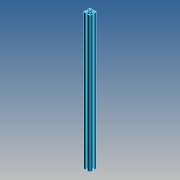
# Autodesk Inventor part: P100
Saved by Autodesk Inventor 2019 (Build 230136000, 136)
## iProperties
Created: 2016-06-02
Part Number: P100
Material: Aluminium
Document SubType Name: Modeling
Designer: serge.amoos
Density: 2.7 g/cm^3
Appearance: Sky Blue Dark
Description: Colonne
Author: serge.amoos
Autodesk Inventor part; units mm, degrees
ref_plane "YZ Plane" through (0, 0, 0) normal (1, 0, 0) x (0, 1, 0)
ref_plane "XZ Plane" through (0, 0, 0) normal (0, 1, 0) x (-1, 0, 0)
ref_plane "XY Plane" through (0, 0, 0) normal (0, 0, 1) x (1, 0, 0)
sketch "Sketch1" plane through (0, 0, 0) normal (0, 0, 1) x (1, 0, 0)
  line L0 (-24, 0) -> (4, 0) construction
  line L1 (0, -4) -> (0, 24) construction
  line L2 (0, 0) -> (-20, 20)
  line L3 (-20, 20) -> (0, 20)
  line L4 (0, 20) -> (0, 0)
  dimension "d0" = 20
  dimension "d1" = 45
  constraints: 6 end point, 1 perpendicular, 1 point on line
  measures "d0" distance of L2.end L3.end
  measures "d1" angle of L1 L2
extrude "Corps" add sketch "Sketch1" along normal blind 800
sketch "Sketch2" plane through (0, 0, 800) normal (0, 0, 1) x (1, 0, 0)
  line L0 (-20, 20) -> (0, 20) construction
  line L1 (0, 20) -> (0, 0) construction
  line L2 (0, 0) -> (-20, 20) construction
  line L3 (-10, 12.1213) -> (-5.3787, 7.5)
  line L4 (-5.3787, 7.5) -> (0, 7.5)
  line L5 (0, 7.5) -> (0, 20)
  line L6 (0, 20) -> (-4, 20)
  line L7 (-4, 20) -> (-4, 15.7)
  line L8 (-4, 15.7) -> (-6, 15.7)
  line L9 (-6, 15.7) -> (-6, 18)
  line L10 (-6, 18) -> (-10, 18)
  line L11 (-10, 18) -> (-10, 12.1213)
  line L12 (-18, 18) -> (-11.5, 18)
  line L13 (-11.5, 18) -> (-11.5, 11.5)
  line L14 (-11.5, 11.5) -> (-18, 18)
  dimension "d4" = 1.5
  dimension "d5" = 4
  dimension "d6" = 2
  dimension "d7" = 4.3
  dimension "d8" = 2
  dimension "d9" = 10
  dimension "d10" = 6.5
  dimension "d12" = 7.5
  constraints: 24 end point, 6 perpendicular, 4 point on line, 3 collinear, 1 horizontal, 1 parallel, 1 vertical
  measures "d4" distance between parallel lines of L2 L3
  measures "d5" distance between parallel lines of L1 L7
  measures "d6" distance between parallel lines of L7 L9
  measures "d7" distance of L6.end L7.end
  measures "d8" distance between parallel lines of L10 L0
  measures "d9" distance from line of L11 L0.start
  measures "d10" distance of L12.start L12.end
  measures "d12" distance from line of L1.end L4
extrude "Creux" cut sketch "Sketch2" against normal through all
fillet "Fillet8" radius 1 1 edges at (-4, 20, 400)
fillet "Fillet1" radius 3 1 edges at (-10, 18, 400)
fillet "Fillet2" radius 1 1 edges at (-6, 18, 400)
fillet "Fillet3" radius 2 2 edges at (-10, 12.1213, 400) (-5.3787, 7.5, 400)
fillet "Fillet4" radius 0.5 2 edges at (-4, 15.7, 400) (-6, 15.7, 400)
fillet "Fillet5" radius 0.5 1 edges at (-11.5, 18, 400)
mirror "Mirror1" about plane through (-20, 20, 0) normal (-0.7071, -0.7071, 0)
fillet "Fillet6" radius 3 1 edges at (-20, 20, 400)
fillet "Fillet7" radius 1 1 edges at (-18, 18, 400)
pattern_circular "Circular Pattern1" count 4 over 360 about axis through (0, 0, 0) along (0, 0, 1)
sketch "Sketch3" plane through (0, 0, 800) normal (0, 0, 1) x (1, 0, 0)
  point P0 (0, 0)
hole "Hole1" at (0, 0, 800) direction (0, 0, -1) diameter 6 end through all
sketch "Sketch4" plane through (0, 0, 800) normal (0, 0, 1) x (1, 0, 0)
  circle A0 centre (0, 0) radius 3 construction
  arc A1 (12, 18) -> (11.5, 17.5) centre (12, 17.5) ccw construction
  line L0 (11.5, 17.5) -> (11.5, 11.5) construction
  line L1 (11.5, 11.5) -> (17.5, 11.5) construction
  arc A2 (17.5, 11.5) -> (18, 12) centre (17.5, 12) ccw construction
  line L2 (18, 12) -> (18, 17) construction
  arc A3 (18, 17) -> (17, 18) centre (17, 17) ccw construction
  line L3 (17, 18) -> (12, 18) construction
  arc A4 (18, -12) -> (17.5, -11.5) centre (17.5, -12) ccw construction
  line L4 (17.5, -11.5) -> (11.5, -11.5) construction
  line L5 (11.5, -11.5) -> (11.5, -17.5) construction
  arc A5 (11.5, -17.5) -> (12, -18) centre (12, -17.5) ccw construction
  line L6 (12, -18) -> (17, -18) construction
  arc A6 (17, -18) -> (18, -17) centre (17, -17) ccw construction
  line L7 (18, -17) -> (18, -12) construction
  arc A7 (-12, -18) -> (-11.5, -17.5) centre (-12, -17.5) ccw construction
  line L8 (-11.5, -17.5) -> (-11.5, -11.5) construction
  line L9 (-11.5, -11.5) -> (-17.5, -11.5) construction
  arc A8 (-17.5, -11.5) -> (-18, -12) centre (-17.5, -12) ccw construction
  line L10 (-18, -12) -> (-18, -17) construction
  arc A9 (-18, -17) -> (-17, -18) centre (-17, -17) ccw construction
  line L11 (-17, -18) -> (-12, -18) construction
  arc A10 (-18, 12) -> (-17.5, 11.5) centre (-17.5, 12) ccw construction
  line L12 (-17.5, 11.5) -> (-11.5, 11.5) construction
  line L13 (-11.5, 11.5) -> (-11.5, 17.5) construction
  arc A11 (-11.5, 17.5) -> (-12, 18) centre (-12, 17.5) ccw construction
  line L14 (-12, 18) -> (-17, 18) construction
  arc A12 (-17, 18) -> (-18, 17) centre (-17, 17) ccw construction
  line L15 (-18, 17) -> (-18, 12) construction
  arc A13 (-6, 17) -> (-7, 18) centre (-7, 17) ccw construction
  arc A14 (-7, 18) -> (-10, 15) centre (-7, 15) ccw construction
  line L16 (-10, 15) -> (-10, 12.9497) construction
  arc A15 (-10, 12.9497) -> (-9.4142, 11.5355) centre (-8, 12.9497) ccw construction
  line L17 (-9.4142, 11.5355) -> (-5.9645, 8.0858) construction
  arc A16 (-5.9645, 8.0858) -> (-4.5503, 7.5) centre (-4.5503, 9.5) ccw construction
  line L18 (-4.5503, 7.5) -> (4.5503, 7.5) construction
  arc A17 (4.5503, 7.5) -> (5.9645, 8.0858) centre (4.5503, 9.5) ccw construction
  line L19 (5.9645, 8.0858) -> (9.4142, 11.5355) construction
  arc A18 (9.4142, 11.5355) -> (10, 12.9497) centre (8, 12.9497) ccw construction
  line L20 (10, 12.9497) -> (10, 15) construction
  arc A19 (10, 15) -> (7, 18) centre (7, 15) ccw construction
  arc A20 (7, 18) -> (6, 17) centre (7, 17) ccw construction
  line L21 (6, 17) -> (6, 16.2) construction
  arc A21 (5.5, 15.7) -> (6, 16.2) centre (5.5, 16.2) ccw construction
  line L22 (5.5, 15.7) -> (4.5, 15.7) construction
  arc A22 (4, 16.2) -> (4.5, 15.7) centre (4.5, 16.2) ccw construction
  line L23 (4, 16.2) -> (4, 19) construction
  arc A23 (5, 20) -> (4, 19) centre (5, 19) ccw construction
  line L24 (5, 20) -> (17, 20) construction
  arc A24 (20, 17) -> (17, 20) centre (17, 17) ccw construction
  line L25 (20, 17) -> (20, 5) construction
  arc A25 (19, 4) -> (20, 5) centre (19, 5) ccw construction
  line L26 (19, 4) -> (16.2, 4) construction
  arc A26 (15.7, 4.5) -> (16.2, 4) centre (16.2, 4.5) ccw construction
  line L27 (15.7, 4.5) -> (15.7, 5.5) construction
  arc A27 (16.2, 6) -> (15.7, 5.5) centre (16.2, 5.5) ccw construction
  line L28 (16.2, 6) -> (17, 6) construction
  arc A28 (17, 6) -> (18, 7) centre (17, 7) ccw construction
  arc A29 (18, 7) -> (15, 10) centre (15, 7) ccw construction
  line L29 (15, 10) -> (12.9497, 10) construction
  arc A30 (12.9497, 10) -> (11.5355, 9.4142) centre (12.9497, 8) ccw construction
  line L30 (11.5355, 9.4142) -> (8.0858, 5.9645) construction
  arc A31 (8.0858, 5.9645) -> (7.5, 4.5503) centre (9.5, 4.5503) ccw construction
  line L31 (7.5, 4.5503) -> (7.5, -4.5503) construction
  arc A32 (7.5, -4.5503) -> (8.0858, -5.9645) centre (9.5, -4.5503) ccw construction
  line L32 (8.0858, -5.9645) -> (11.5355, -9.4142) construction
  arc A33 (11.5355, -9.4142) -> (12.9497, -10) centre (12.9497, -8) ccw construction
  line L33 (12.9497, -10) -> (15, -10) construction
  arc A34 (15, -10) -> (18, -7) centre (15, -7) ccw construction
  arc A35 (18, -7) -> (17, -6) centre (17, -7) ccw construction
  line L34 (17, -6) -> (16.2, -6) construction
  arc A36 (15.7, -5.5) -> (16.2, -6) centre (16.2, -5.5) ccw construction
  line L35 (15.7, -5.5) -> (15.7, -4.5) construction
  arc A37 (16.2, -4) -> (15.7, -4.5) centre (16.2, -4.5) ccw construction
  line L36 (16.2, -4) -> (19, -4) construction
  arc A38 (20, -5) -> (19, -4) centre (19, -5) ccw construction
  line L37 (20, -5) -> (20, -17) construction
  arc A39 (17, -20) -> (20, -17) centre (17, -17) ccw construction
  line L38 (17, -20) -> (5, -20) construction
  arc A40 (4, -19) -> (5, -20) centre (5, -19) ccw construction
  line L39 (4, -19) -> (4, -16.2) construction
  arc A41 (4.5, -15.7) -> (4, -16.2) centre (4.5, -16.2) ccw construction
  line L40 (4.5, -15.7) -> (5.5, -15.7) construction
  arc A42 (6, -16.2) -> (5.5, -15.7) centre (5.5, -16.2) ccw construction
  line L41 (6, -16.2) -> (6, -17) construction
  arc A43 (6, -17) -> (7, -18) centre (7, -17) ccw construction
  arc A44 (7, -18) -> (10, -15) centre (7, -15) ccw construction
  line L42 (10, -15) -> (10, -12.9497) construction
  arc A45 (10, -12.9497) -> (9.4142, -11.5355) centre (8, -12.9497) ccw construction
  line L43 (9.4142, -11.5355) -> (5.9645, -8.0858) construction
  arc A46 (5.9645, -8.0858) -> (4.5503, -7.5) centre (4.5503, -9.5) ccw construction
  line L44 (4.5503, -7.5) -> (-4.5503, -7.5) construction
  arc A47 (-4.5503, -7.5) -> (-5.9645, -8.0858) centre (-4.5503, -9.5) ccw construction
  line L45 (-5.9645, -8.0858) -> (-9.4142, -11.5355) construction
  arc A48 (-9.4142, -11.5355) -> (-10, -12.9497) centre (-8, -12.9497) ccw construction
  line L46 (-10, -12.9497) -> (-10, -15) construction
  arc A49 (-10, -15) -> (-7, -18) centre (-7, -15) ccw construction
  arc A50 (-7, -18) -> (-6, -17) centre (-7, -17) ccw construction
  line L47 (-6, -17) -> (-6, -16.2) construction
  arc A51 (-5.5, -15.7) -> (-6, -16.2) centre (-5.5, -16.2) ccw construction
  line L48 (-5.5, -15.7) -> (-4.5, -15.7) construction
  arc A52 (-4, -16.2) -> (-4.5, -15.7) centre (-4.5, -16.2) ccw construction
  line L49 (-4, -16.2) -> (-4, -19) construction
  arc A53 (-5, -20) -> (-4, -19) centre (-5, -19) ccw construction
  line L50 (-5, -20) -> (-17, -20) construction
  arc A54 (-20, -17) -> (-17, -20) centre (-17, -17) ccw construction
  line L51 (-20, -17) -> (-20, -5) construction
  arc A55 (-19, -4) -> (-20, -5) centre (-19, -5) ccw construction
  line L52 (-19, -4) -> (-16.2, -4) construction
  arc A56 (-15.7, -4.5) -> (-16.2, -4) centre (-16.2, -4.5) ccw construction
  line L53 (-15.7, -4.5) -> (-15.7, -5.5) construction
  arc A57 (-16.2, -6) -> (-15.7, -5.5) centre (-16.2, -5.5) ccw construction
  line L54 (-16.2, -6) -> (-17, -6) construction
  arc A58 (-17, -6) -> (-18, -7) centre (-17, -7) ccw construction
  arc A59 (-18, -7) -> (-15, -10) centre (-15, -7) ccw construction
  line L55 (-15, -10) -> (-12.9497, -10) construction
  arc A60 (-12.9497, -10) -> (-11.5355, -9.4142) centre (-12.9497, -8) ccw construction
  line L56 (-11.5355, -9.4142) -> (-8.0858, -5.9645) construction
  arc A61 (-8.0858, -5.9645) -> (-7.5, -4.5503) centre (-9.5, -4.5503) ccw construction
  line L57 (-7.5, -4.5503) -> (-7.5, 4.5503) construction
  arc A62 (-7.5, 4.5503) -> (-8.0858, 5.9645) centre (-9.5, 4.5503) ccw construction
  line L58 (-8.0858, 5.9645) -> (-11.5355, 9.4142) construction
  arc A63 (-11.5355, 9.4142) -> (-12.9497, 10) centre (-12.9497, 8) ccw construction
  line L59 (-12.9497, 10) -> (-15, 10) construction
  arc A64 (-15, 10) -> (-18, 7) centre (-15, 7) ccw construction
  arc A65 (-18, 7) -> (-17, 6) centre (-17, 7) ccw construction
  line L60 (-17, 6) -> (-16.2, 6) construction
  arc A66 (-15.7, 5.5) -> (-16.2, 6) centre (-16.2, 5.5) ccw construction
  line L61 (-15.7, 5.5) -> (-15.7, 4.5) construction
  arc A67 (-16.2, 4) -> (-15.7, 4.5) centre (-16.2, 4.5) ccw construction
  line L62 (-16.2, 4) -> (-19, 4) construction
  arc A68 (-20, 5) -> (-19, 4) centre (-19, 5) ccw construction
  line L63 (-20, 5) -> (-20, 17) construction
  arc A69 (-17, 20) -> (-20, 17) centre (-17, 17) ccw construction
  line L64 (-17, 20) -> (-5, 20) construction
  arc A70 (-4, 19) -> (-5, 20) centre (-5, 19) ccw construction
  line L65 (-4, 19) -> (-4, 16.2) construction
  arc A71 (-4.5, 15.7) -> (-4, 16.2) centre (-4.5, 16.2) ccw construction
  line L66 (-4.5, 15.7) -> (-5.5, 15.7) construction
  arc A72 (-6, 16.2) -> (-5.5, 15.7) centre (-5.5, 16.2) ccw construction
  line L67 (-6, 16.2) -> (-6, 17) construction
  line L68 (-9.5, 20) -> (12.6978, 20)
  line L69 (12.6978, 20) -> (12.6978, 18)
  line L70 (12.6978, 18) -> (-9.5, 18)
  line L71 (-9.5, 18) -> (-9.5, 20)
  constraints: 8 end point, 2 parallel, 2 point on line, 1 horizontal, 1 perpendicular
extrude "Extrusion4" add sketch "Sketch4" against normal blind 800
body "Solid1"
